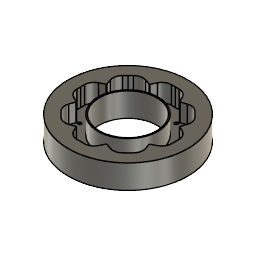
Nisip_Ghiveci (Autodesk Fusion 360 design; units mm, degrees)
part number: 2026-06-05-19-29-36-104
Autodesk Fusion 360 part; units mm, degrees
sketch "Sketch1" plane through (0, 0, 0) normal (0, 0, 1) x (1, 0, 0)
  arc A0 (13, 11.1068) -> (11.8, 12.3068) centre (11.8, 11.1068) ccw
  arc A1 (3.223, 0) -> (10.4161, 4.4986) centre (3.223, 8) ccw
  arc A2 (3.223, 0) -> (10.4161, 4.4986) centre (3.223, 8) ccw
  line L0 (10.5, 9.8068) -> (10.4144, 9.8073)
  arc A3 (13, 11.1068) -> (11.8, 12.3068) centre (11.8, 11.1068) ccw
  line L1 (10.5, 12.3068) -> (11.8, 12.3068)
  line L2 (10.5, 12.3068) -> (11.8, 12.3068)
  line L3 (13, 11.1068) -> (13, 10.9591)
  line L4 (13, 11.1068) -> (13, 10.9591)
  line L5 (12.4957, 8.7708) -> (10.4161, 4.4986)
  line L6 (10.2599, 10.1289) -> (10.5, 9.8068)
  line L7 (12.4957, 8.7708) -> (10.4161, 4.4986)
  arc A4 (12.4957, 8.7708) -> (13, 10.9591) centre (8, 10.9591) ccw
  line L8 (10.5, 12.3068) -> (-10.5, 12.3068)
  line L9 (0, 0) -> (3.223, 0)
  arc A5 (-13, 10.9591) -> (-12.4957, 8.7708) centre (-8, 10.9591) ccw
  line L10 (0, 0) -> (3.223, 0)
  line L11 (-12.4957, 8.7708) -> (-10.4161, 4.4986)
  line L12 (-3.223, 0) -> (0, 0)
  line L13 (-13, 11.1068) -> (-13, 10.9591)
  line L14 (-10.5, 12.3068) -> (-11.8, 12.3068)
  arc A6 (-11.8, 12.3068) -> (-13, 11.1068) centre (-11.8, 11.1068) ccw
  arc A7 (-10.4161, 4.4986) -> (-3.223, 0) centre (-3.223, 8) ccw
  arc A8 (12.4957, 8.7708) -> (13, 10.9591) centre (8, 10.9591) ccw
  circle A9 centre (-11.8, 11.1068) radius 0.875
  circle A10 centre (11.8, 11.1068) radius 0.875
  point P0 (-13, 12.3068)
  point P1 (13, 12.3068)
  dimension "d18" = 2.5
  dimension "d19" = 2.5
  dimension "d20" = 1.2
  dimension "d21" = 5
  dimension "d22" = 8
  dimension "d25" = 115.956
  dimension "d26" = 1.2
  dimension "d27" = 5
  dimension "d28" = 8
  dimension "d30" = 115.956
  dimension "d34" = 10.4144
  dimension "d35" = 9.8073
  dimension "d36" = 12.3068
  dimension "d37" = 13
  dimension "d38" = 13
  dimension "d39" = 8
  dimension "d40" = 12.3068
  dimension "d41" = 117.339
  dimension "d42" = 115.956
  dimension "d43" = 0.322
  dimension "d44" = 1.3477
  dimension "d45" = 1.75
  dimension "d46" = 1.75
  constraint horizontal L2
  constraint vertical L4
  constraint coincident L1.start L2.start
  constraint coincident L9.start L10.start
  constraint coincident P1 L2
  constraint coincident P1 L4
  constraint tangent A3 L2
  constraint tangent A3 L4
  constraint tangent L4 A4
  constraint tangent L5 A4
  constraint tangent A2 L9
  constraint tangent A2 L5
  constraint tangent A5 L13
  constraint tangent A5 L11
  constraint tangent L13 A6
  constraint tangent L14 A6
  constraint equal A4 A5
  constraint equal A3 A6
  constraint tangent L11 A7
  constraint tangent L12 A7
  constraint equal A2 A7
  constraint equal L4 L13
  constraint equal L2 L14
  constraint horizontal L8.end P0
  constraint collinear L2 L14
  constraint equal L9 L12
  constraint equal L5 L11
  constraint horizontal L1
  constraint vertical L3
  constraint tangent A0 L1
  constraint tangent A0 L3
  constraint tangent L3 A8
  constraint tangent L7 A8
  constraint tangent A1 L10
  constraint tangent A1 L7
  constraint tangent A1 L9
  constraint tangent A1 L5
  constraint tangent A0 L2
  constraint tangent L5 A8
  constraint tangent L4 A8
  constraint tangent A1 A2
  constraint collinear L5 L7
  constraint vertical L1.start L0.start
  constraint coincident L8.end L14.start
  constraint vertical P0 L13.start
  constraint concentric A6 A9
  constraint concentric A3 A10
  measures "d18" distance of L1.start P1
  measures "d19" distance of L1.start L0.start
  measures "d20" radius of A3
  measures "d21" radius of A4
  measures "d22" radius of A2
  measures "d25" angle of L5 L9
  measures "d26" radius of A0
  measures "d27" radius of A8
  measures "d28" radius of A1
  measures "d30" angle of L7 L10
  measures "d34" horizontal distance of L9.start L0.end
  measures "d35" vertical distance of L9.start L0.end
  measures "d36" distance of L9.start L8
  measures "d37" distance of L9.start L13
  measures "d38" distance of L9.start L4
  measures "d39" vertical distance of L9.start A1.centre
  measures "d40" distance of L9 L14
  measures "d41" angle of L5 L6
  measures "d42" angle of L11 L12
  measures "d43" vertical distance of L0.start L6.start
  measures "d44" distance of A4.centre L8
  measures "d45" diameter of A9
  measures "d46" diameter of A10
sketch "Sketch2" plane through (0, 0, 0) normal (0, 0, 1) x (1, 0, 0)
  line L0 (12.953, 8.964) -> (17.4443, 7.4136)
  circle A0 centre (11.793, 11.1078) radius 0.875
  line L1 (11.8637, 12.8755) -> (10.9445, 11.9563)
  arc A1 (17.4443, 7.4136) -> (25.7116, 9.3189) centre (20.0547, 14.9758) ccw
  arc A2 (10.9445, 11.9563) -> (10.9445, 10.2593) centre (11.793, 11.1078) ccw
  arc A3 (11.0489, 10.1548) -> (12.953, 8.964) centre (14.5845, 13.6903) ccw
  line L2 (27.9906, 11.5979) -> (30.2696, 13.877)
  line L3 (10.9445, 10.2593) -> (11.0489, 10.1548)
  circle A4 centre (28.4807, 27.7955) radius 0.875
  line L4 (27.9906, 11.5979) -> (30.2696, 13.877)
  arc A5 (30.6245, 26.6356) -> (29.4337, 28.5396) centre (25.8982, 25.0041) ccw
  line L5 (26.713, 27.7248) -> (27.6322, 28.644)
  arc A6 (30.2696, 13.877) -> (32.1749, 22.1442) centre (24.6128, 19.5338) ccw
  line L6 (25.7116, 9.3189) -> (27.9906, 11.5979)
  arc A7 (30.2696, 13.877) -> (32.1749, 22.1442) centre (24.6128, 19.5338) ccw
  arc A8 (30.6245, 26.6356) -> (29.4337, 28.5396) centre (25.8982, 25.0041) ccw
  line L7 (28.0833, 26.015) -> (28.4807, 25.957)
  line L8 (29.3293, 28.644) -> (29.4337, 28.5396)
  line L9 (29.3293, 28.644) -> (29.4337, 28.5396)
  arc A9 (29.3293, 28.644) -> (27.6322, 28.644) centre (28.4807, 27.7955) ccw
  line L10 (26.713, 27.7248) -> (11.8637, 12.8755)
  line L11 (26.713, 27.7248) -> (27.6322, 28.644)
  line L12 (30.6245, 26.6356) -> (32.1749, 22.1442)
  line L13 (28.4807, 25.957) -> (28.4199, 25.8969)
  arc A10 (29.3293, 28.644) -> (27.6322, 28.644) centre (28.4807, 27.7955) ccw
  line L14 (30.6245, 26.6356) -> (32.1749, 22.1442)
  line L15 (30.8154, 27.1043) -> (35.0875, 29.1838)
  circle A11 centre (28.4793, 27.7999) radius 0.875
  line L16 (27.2793, 29.0999) -> (27.2793, 27.7999)
  arc A12 (35.0875, 29.1838) -> (39.5861, 36.3769) centre (31.5861, 36.3769) ccw
  arc A13 (27.2793, 27.7999) -> (28.4793, 26.5999) centre (28.4793, 27.7999) ccw
  arc A14 (28.627, 26.5999) -> (30.8154, 27.1043) centre (28.627, 31.5999) ccw
  line L17 (39.5861, 39.5999) -> (39.5861, 42.823)
  line L18 (28.4793, 26.5999) -> (28.627, 26.5999)
  circle A15 centre (28.4793, 51.3999) radius 0.875
  line L19 (39.5861, 39.5999) -> (39.5861, 42.823)
  arc A16 (30.8154, 52.0956) -> (28.627, 52.5999) centre (28.627, 47.5999) ccw
  line L20 (27.2793, 50.0999) -> (27.2793, 51.3999)
  arc A17 (39.5861, 42.823) -> (35.0875, 50.0161) centre (31.5861, 42.823) ccw
  line L21 (39.5861, 36.3769) -> (39.5861, 39.5999)
  arc A18 (39.5861, 42.823) -> (35.0875, 50.0161) centre (31.5861, 42.823) ccw
  arc A19 (30.8154, 52.0956) -> (28.627, 52.5999) centre (28.627, 47.5999) ccw
  line L22 (29.4573, 49.8599) -> (29.7793, 50.0999)
  line L23 (28.4793, 52.5999) -> (28.627, 52.5999)
  line L24 (28.4793, 52.5999) -> (28.627, 52.5999)
  arc A20 (28.4793, 52.5999) -> (27.2793, 51.3999) centre (28.4793, 51.3999) ccw
  line L25 (27.2793, 50.0999) -> (27.2793, 29.0999)
  line L26 (27.2793, 50.0999) -> (27.2793, 51.3999)
  line L27 (30.8154, 52.0956) -> (35.0875, 50.0161)
  line L28 (29.7793, 50.0999) -> (29.7788, 50.0144)
  arc A21 (28.4793, 52.5999) -> (27.2793, 51.3999) centre (28.4793, 51.3999) ccw
  line L29 (30.8154, 52.0956) -> (35.0875, 50.0161)
  line L30 (3.1934, 79.2434) -> (-0.0296, 79.2434)
  line L31 (-10.5296, 66.9366) -> (-11.8296, 66.9366)
  line L32 (-10.5296, 66.9366) -> (10.4704, 66.9366)
  arc A22 (-3.2527, 79.2434) -> (-10.4458, 74.7448) centre (-3.2527, 71.2434) ccw
  arc A23 (-13.0296, 68.1366) -> (-11.8296, 66.9366) centre (-11.8296, 68.1366) ccw
  line L33 (-12.5253, 70.4727) -> (-10.4458, 74.7448)
  line L34 (-13.0296, 68.1366) -> (-13.0296, 68.2843)
  arc A24 (-12.5253, 70.4727) -> (-13.0296, 68.2843) centre (-8.0296, 68.2843) ccw
  line L35 (11.8455, 66.3703) -> (10.9263, 67.2895)
  line L36 (13.5553, 67.7406) -> (13.6133, 68.1381)
  arc A25 (10.9263, 68.9866) -> (10.9263, 67.2895) centre (11.7748, 68.1381) ccw
  arc A26 (25.6933, 69.9269) -> (17.4261, 71.8322) centre (20.0365, 64.2701) ccw
  line L37 (13.6133, 68.1381) -> (13.6734, 68.0772)
  line L38 (10.9263, 68.9866) -> (11.0307, 69.091)
  arc A27 (11.7704, 66.9366) -> (12.9704, 68.1366) centre (11.7704, 68.1366) ccw
  line L39 (12.466, 70.4727) -> (10.3865, 74.7448)
  line L40 (11.8455, 66.3703) -> (10.9263, 67.2895)
  arc A28 (12.9704, 68.2843) -> (12.466, 70.4727) centre (7.9704, 68.2843) ccw
  arc A29 (10.3865, 74.7448) -> (3.1934, 79.2434) centre (3.1934, 71.2434) ccw
  line L41 (10.4704, 66.9366) -> (11.7704, 66.9366)
  line L42 (12.9347, 70.2818) -> (17.4261, 71.8322)
  arc A30 (25.6933, 69.9269) -> (17.4261, 71.8322) centre (20.0365, 64.2701) ccw
  circle A31 centre (11.7748, 68.1381) radius 0.875
  circle A32 centre (11.7704, 68.1366) radius 0.875
  arc A33 (12.9347, 70.2818) -> (11.0307, 69.091) centre (14.5663, 65.5555) ccw
  line L43 (-0.0296, 79.2434) -> (-3.2527, 79.2434)
  arc A34 (-3.2527, 79.2434) -> (-10.4458, 74.7448) centre (-3.2527, 71.2434) ccw
  circle A35 centre (-11.8296, 68.1366) radius 0.875
  line L44 (27.9724, 67.6479) -> (25.6933, 69.9269)
  line L45 (11.8455, 66.3703) -> (26.6948, 51.521)
  circle A36 centre (28.4625, 51.4503) radius 0.875
  arc A37 (32.1567, 57.1016) -> (30.2514, 65.3689) centre (24.5945, 59.712) ccw
  arc A38 (29.4155, 50.7062) -> (30.6063, 52.6103) centre (25.88, 54.2418) ccw
  line L46 (27.9724, 67.6479) -> (25.6933, 69.9269)
  line L47 (26.6948, 51.521) -> (27.614, 50.6018)
  arc A39 (27.614, 50.6018) -> (29.3111, 50.6018) centre (28.4625, 51.4503) ccw
  line L48 (30.6063, 52.6103) -> (32.1567, 57.1016)
  arc A40 (12.9347, 70.2818) -> (11.0307, 69.091) centre (14.5663, 65.5555) ccw
  arc A41 (10.9263, 68.9866) -> (10.9263, 67.2895) centre (11.7748, 68.1381) ccw
  line L49 (12.9347, 70.2818) -> (17.4261, 71.8322)
  line L50 (12.9704, 68.1366) -> (12.9704, 68.2843)
  line L51 (10.9263, 68.9866) -> (11.0307, 69.091)
  line L52 (-12.5253, 70.4727) -> (-10.4458, 74.7448)
  arc A42 (-12.5253, 70.4727) -> (-13.0296, 68.2843) centre (-8.0296, 68.2843) ccw
  line L53 (-10.5296, 69.4366) -> (-10.4441, 69.4361)
  line L54 (-0.0296, 79.2434) -> (-3.2527, 79.2434)
  arc A43 (-13.0296, 68.1366) -> (-11.8296, 66.9366) centre (-11.8296, 68.1366) ccw
  line L55 (-10.5296, 66.9366) -> (-11.8296, 66.9366)
  line L56 (29.3111, 50.6018) -> (29.4155, 50.7062)
  line L57 (30.2514, 65.3689) -> (27.9724, 67.6479)
  line L58 (-13.0296, 68.1366) -> (-13.0296, 68.2843)
  line L59 (-10.2896, 69.1146) -> (-10.5296, 69.4366)
  line L60 (12.9689, 11.1314) -> (12.9689, 10.9837)
  line L61 (12.9689, 11.1314) -> (12.9689, 10.9837)
  line L62 (-0.0311, 0.0246) -> (3.192, 0.0246)
  arc A44 (12.4646, 8.7953) -> (12.9689, 10.9837) centre (7.9689, 10.9837) ccw
  line L63 (12.4646, 8.7953) -> (10.385, 4.5232)
  arc A45 (12.9689, 11.1314) -> (11.7689, 12.3314) centre (11.7689, 11.1314) ccw
  line L64 (10.4689, 9.8314) -> (10.3834, 9.8319)
  line L65 (10.4689, 12.3314) -> (11.7689, 12.3314)
  arc A46 (3.192, 0.0246) -> (10.385, 4.5232) centre (3.192, 8.0246) ccw
  line L66 (-11.9244, 66.3925) -> (-11.0052, 67.3117)
  arc A47 (-11.1097, 69.1132) -> (-13.0137, 70.304) centre (-14.6452, 65.5777) ccw
  line L67 (10.4689, 12.3314) -> (-10.5311, 12.3314)
  arc A48 (-11.0052, 67.3117) -> (-11.0052, 69.0088) centre (-11.8537, 68.1602) ccw
  line L68 (-11.0052, 69.0088) -> (-11.1097, 69.1132)
  arc A49 (-10.4472, 4.5232) -> (-3.2541, 0.0246) centre (-3.2541, 8.0246) ccw
  line L69 (-28.0513, 67.6701) -> (-30.3303, 65.3911)
  line L70 (-28.0513, 67.6701) -> (-30.3303, 65.3911)
  line L71 (-26.7737, 51.5432) -> (-11.9244, 66.3925)
  line L72 (10.4689, 12.3314) -> (11.7689, 12.3314)
  line L73 (-3.2541, 0.0246) -> (-0.0311, 0.0246)
  arc A50 (3.192, 0.0246) -> (10.385, 4.5232) centre (3.192, 8.0246) ccw
  circle A51 centre (11.7689, 11.1314) radius 0.875
  line L74 (-11.9062, 12.8977) -> (-10.987, 11.9785)
  line L75 (-13.616, 11.5274) -> (-13.674, 11.13)
  arc A52 (-12.9955, 8.9862) -> (-11.0914, 10.177) centre (-14.627, 13.7125) ccw
  line L76 (-10.987, 10.2814) -> (-11.0914, 10.177)
  arc A53 (-11.8311, 12.3314) -> (-13.0311, 11.1314) centre (-11.8311, 11.1314) ccw
  arc A54 (-13.0311, 10.9837) -> (-12.5267, 8.7953) centre (-8.0311, 10.9837) ccw
  arc A55 (-12.9955, 8.9862) -> (-11.0914, 10.177) centre (-14.627, 13.7125) ccw
  arc A56 (-25.7541, 9.3411) -> (-17.4868, 7.4358) centre (-20.0972, 14.9979) ccw
  line L77 (-10.5311, 12.3314) -> (-11.8311, 12.3314)
  line L78 (-12.9955, 8.9862) -> (-17.4868, 7.4358)
  arc A57 (-10.987, 10.2814) -> (-10.987, 11.9785) centre (-11.8355, 11.13) ccw
  arc A58 (-10.987, 10.2814) -> (-10.987, 11.9785) centre (-11.8355, 11.13) ccw
  line L79 (-12.9955, 8.9862) -> (-17.4868, 7.4358)
  line L80 (-10.987, 10.2814) -> (-11.0914, 10.177)
  line L81 (-39.6468, 39.6681) -> (-39.6468, 36.445)
  line L82 (-26.7555, 27.747) -> (-27.6747, 28.6662)
  line L83 (-29.84, 29.1681) -> (-29.8395, 29.2536)
  line L84 (-30.3121, 13.8991) -> (-28.0331, 11.6201)
  line L85 (-29.3718, 28.6662) -> (-29.4762, 28.5618)
  arc A59 (-32.2174, 22.1664) -> (-30.3121, 13.8991) centre (-24.6553, 19.556) ccw
  arc A60 (-30.8761, 27.1724) -> (-28.6877, 26.6681) centre (-28.6877, 31.6681) ccw
  arc A61 (-39.6468, 36.445) -> (-35.1482, 29.252) centre (-31.6468, 36.445) ccw
  circle A62 centre (-28.5232, 27.8177) radius 0.875
  line L86 (-30.667, 26.6577) -> (-32.2174, 22.1664)
  arc A63 (-29.4762, 28.5618) -> (-30.667, 26.6577) centre (-25.9407, 25.0262) ccw
  arc A64 (-27.6747, 28.6662) -> (-29.3718, 28.6662) centre (-28.5232, 27.8177) ccw
  line L87 (-27.34, 29.1681) -> (-27.34, 27.8681)
  circle A65 centre (-11.8311, 11.1314) radius 0.875
  circle A66 centre (-11.8537, 68.1602) radius 0.875
  line L88 (-25.7723, 69.9491) -> (-28.0513, 67.6701)
  line L89 (-30.6852, 52.6325) -> (-32.2356, 57.1238)
  line L90 (-39.6468, 42.8911) -> (-39.6468, 39.6681)
  arc A67 (-17.505, 71.8544) -> (-25.7723, 69.9491) centre (-20.1154, 64.2923) ccw
  line L91 (-13.0137, 70.304) -> (-17.505, 71.8544)
  line L92 (-27.34, 29.1681) -> (-27.34, 50.1681)
  arc A68 (12.9689, 11.1314) -> (11.7689, 12.3314) centre (11.7689, 11.1314) ccw
  line L93 (12.4646, 8.7953) -> (10.385, 4.5232)
  arc A69 (12.4646, 8.7953) -> (12.9689, 10.9837) centre (7.9689, 10.9837) ccw
  line L94 (-0.0311, 0.0246) -> (3.192, 0.0246)
  line L95 (10.2288, 10.1534) -> (10.4689, 9.8314)
  arc A70 (-30.3303, 65.3911) -> (-32.2356, 57.1238) centre (-24.6735, 59.7342) ccw
  line L96 (-28.54, 52.6681) -> (-28.6877, 52.6681)
  line L97 (-28.144, 53.253) -> (-28.5415, 53.311)
  line L98 (-30.6852, 52.6325) -> (-32.2356, 57.1238)
  line L99 (-28.5415, 53.311) -> (-28.4806, 53.3711)
  arc A71 (-30.3303, 65.3911) -> (-32.2356, 57.1238) centre (-24.6735, 59.7342) ccw
  arc A72 (-35.1482, 50.0842) -> (-39.6468, 42.8911) centre (-31.6468, 42.8911) ccw
  line L100 (-29.39, 50.624) -> (-29.4944, 50.7284)
  line L101 (-27.34, 50.1681) -> (-27.34, 51.4681)
  line L102 (-26.7737, 51.5432) -> (-27.6929, 50.624)
  arc A73 (-30.6852, 52.6325) -> (-29.4944, 50.7284) centre (-25.9589, 54.264) ccw
  circle A74 centre (-28.54, 51.4681) radius 0.875
  arc A75 (-25.7541, 9.3411) -> (-17.4868, 7.4358) centre (-20.0972, 14.9979) ccw
  line L103 (-11.9062, 12.8977) -> (-10.987, 11.9785)
  line L104 (-13.674, 11.13) -> (-13.7341, 11.1908)
  circle A76 centre (-11.8355, 11.13) radius 0.875
  line L105 (-13.0311, 11.1314) -> (-13.0311, 10.9837)
  line L106 (-12.5267, 8.7953) -> (-10.4472, 4.5232)
  circle A77 centre (-28.54, 27.8681) radius 0.875
  arc A78 (-28.54, 26.6681) -> (-27.34, 27.8681) centre (-28.54, 27.8681) ccw
  arc A79 (-39.6468, 36.445) -> (-35.1482, 29.252) centre (-31.6468, 36.445) ccw
  line L107 (-28.0331, 11.6201) -> (-25.7541, 9.3411)
  line L108 (-30.8761, 27.1724) -> (-35.1482, 29.252)
  circle A80 centre (-28.5415, 51.4725) radius 0.875
  arc A81 (-29.39, 50.624) -> (-27.6929, 50.624) centre (-28.5415, 51.4725) ccw
  line L109 (-30.8761, 52.1637) -> (-35.1482, 50.0842)
  line L110 (-28.54, 26.6681) -> (-28.6877, 26.6681)
  line L111 (-29.39, 50.624) -> (-29.4944, 50.7284)
  line L112 (-30.8761, 27.1724) -> (-35.1482, 29.252)
  arc A82 (-28.54, 26.6681) -> (-27.34, 27.8681) centre (-28.54, 27.8681) ccw
  line L113 (-29.518, 29.4082) -> (-29.84, 29.1681)
  arc A83 (-28.6877, 52.6681) -> (-30.8761, 52.1637) centre (-28.6877, 47.6681) ccw
  arc A84 (-30.8761, 27.1724) -> (-28.6877, 26.6681) centre (-28.6877, 31.6681) ccw
  line L114 (-28.54, 26.6681) -> (-28.6877, 26.6681)
  line L115 (-26.7737, 51.5432) -> (-27.6929, 50.624)
  line L116 (-28.0331, 11.6201) -> (-25.7541, 9.3411)
  line L117 (-11.9062, 12.8977) -> (-26.7555, 27.747)
  arc A85 (-27.34, 51.4681) -> (-28.54, 52.6681) centre (-28.54, 51.4681) ccw
  arc A86 (-30.6852, 52.6325) -> (-29.4944, 50.7284) centre (-25.9589, 54.264) ccw
  line L118 (-39.6468, 39.6681) -> (-39.6468, 36.445)
  arc A87 (-29.39, 50.624) -> (-27.6929, 50.624) centre (-28.5415, 51.4725) ccw
  line L119 (-27.34, 29.1681) -> (-27.34, 27.8681)
  line L120 (11.2792, 66.9366) -> (-11.3399, 12.3314)
  line L121 (-11.3399, 12.3314) -> (-11.3316, 12.3514)
  line L122 (11.3196, 12.3314) -> (-11.3803, 66.9366)
  circle A88 centre (-0.0304, 39.634) radius 25
  circle A89 centre (-0.0304, 39.634) radius 50
  circle A90 centre (-0.0304, 39.634) radius 24
  point P0 (27.9906, 11.5979)
  point P1 (10.096, 11.1078)
  point P2 (28.4807, 29.4926)
  point P3 (27.9906, 11.5979)
  point P4 (39.5861, 39.5999)
  point P5 (27.2793, 26.5999)
  point P6 (27.2793, 52.5999)
  point P7 (39.5861, 39.5999)
  point P8 (-13.0296, 66.9366)
  point P9 (-0.0296, 79.2434)
  point P10 (-0.0296, 79.2434)
  point P11 (12.9704, 66.9366)
  point P12 (27.9724, 67.6479)
  point P13 (28.4625, 49.7533)
  point P14 (27.9724, 67.6479)
  point P15 (10.0777, 68.1381)
  point P16 (-28.5232, 29.5147)
  point P17 (-28.0331, 11.6201)
  point P18 (-10.1385, 11.13)
  point P19 (-28.0331, 11.6201)
  point P20 (-27.34, 26.6681)
  point P21 (-39.6468, 39.6681)
  point P22 (-39.6468, 39.6681)
  point P23 (-27.34, 52.6681)
  point P24 (-0.0607, 79.268)
  point P25 (-28.0513, 67.6701)
  point P26 (-10.1567, 68.1602)
  point P27 (-28.0513, 67.6701)
  point P28 (-28.5415, 49.7755)
  point P29 (12.9689, 12.3314)
  point P30 (-0.0311, 0.0246)
  point P31 (-0.0311, 0.0246)
  point P32 (-13.0311, 12.3314)
  dimension "d49" = 2.5
  dimension "d50" = 2.5
  dimension "d51" = 1.2
  dimension "d52" = 5
  dimension "d53" = 8
  dimension "d54" = 115.956
  dimension "d55" = 1.2
  dimension "d56" = 5
  dimension "d57" = 8
  dimension "d58" = 115.956
  dimension "d61" = 12.3068
  dimension "d62" = 13
  dimension "d63" = 13
  dimension "d65" = 12.3068
  dimension "d66" = 117.339
  dimension "d67" = 115.956
  dimension "d69" = 1.3477
  dimension "d70" = 1.75
  dimension "d71" = 1.75
  dimension "d72" = 2.5
  dimension "d73" = 2.5
  dimension "d74" = 1.2
  dimension "d75" = 5
  dimension "d76" = 8
  dimension "d77" = 115.956
  dimension "d78" = 1.2
  dimension "d79" = 5
  dimension "d80" = 8
  dimension "d81" = 115.956
  dimension "d84" = 12.3068
  dimension "d85" = 13
  dimension "d86" = 13
  dimension "d88" = 12.3068
  dimension "d89" = 117.339
  dimension "d90" = 115.956
  dimension "d92" = 1.3477
  dimension "d93" = 1.75
  dimension "d94" = 1.75
  dimension "d95" = 2.5
  dimension "d96" = 2.5
  dimension "d97" = 1.2
  dimension "d98" = 5
  dimension "d99" = 8
  dimension "d100" = 115.956
  dimension "d101" = 1.2
  dimension "d102" = 5
  dimension "d103" = 8
  dimension "d104" = 115.956
  dimension "d105" = 12.3068
  dimension "d106" = 13
  dimension "d107" = 13
  dimension "d108" = 12.3068
  dimension "d109" = 117.339
  dimension "d110" = 115.956
  dimension "d111" = 1.3477
  dimension "d112" = 1.75
  dimension "d113" = 1.75
  dimension "d114" = 2.5
  dimension "d115" = 2.5
  dimension "d116" = 1.2
  dimension "d117" = 5
  dimension "d118" = 8
  dimension "d119" = 115.956
  dimension "d120" = 1.2
  dimension "d121" = 5
  dimension "d122" = 8
  dimension "d123" = 115.956
  dimension "d124" = 12.3068
  dimension "d125" = 13
  dimension "d126" = 13
  dimension "d127" = 12.3068
  dimension "d128" = 117.339
  dimension "d129" = 115.956
  dimension "d130" = 1.3477
  dimension "d131" = 1.75
  dimension "d132" = 1.75
  dimension "d133" = 2.5
  dimension "d134" = 2.5
  dimension "d135" = 1.2
  dimension "d136" = 5
  dimension "d137" = 8
  dimension "d138" = 115.956
  dimension "d139" = 1.2
  dimension "d140" = 5
  dimension "d141" = 8
  dimension "d142" = 115.956
  dimension "d143" = 12.3068
  dimension "d144" = 13
  dimension "d145" = 13
  dimension "d146" = 12.3068
  dimension "d147" = 117.339
  dimension "d148" = 115.956
  dimension "d149" = 1.3477
  dimension "d150" = 1.75
  dimension "d151" = 1.75
  dimension "d152" = 2.5
  dimension "d153" = 2.5
  dimension "d154" = 1.2
  dimension "d155" = 5
  dimension "d156" = 8
  dimension "d157" = 115.956
  dimension "d158" = 1.2
  dimension "d159" = 5
  dimension "d160" = 8
  dimension "d161" = 115.956
  dimension "d162" = 12.3068
  dimension "d163" = 13
  dimension "d164" = 13
  dimension "d165" = 12.3068
  dimension "d166" = 117.339
  dimension "d167" = 115.956
  dimension "d168" = 1.3477
  dimension "d169" = 1.75
  dimension "d170" = 1.75
  dimension "d171" = 2.5
  dimension "d172" = 2.5
  dimension "d173" = 1.2
  dimension "d174" = 5
  dimension "d175" = 8
  dimension "d176" = 115.956
  dimension "d177" = 1.2
  dimension "d178" = 5
  dimension "d179" = 8
  dimension "d180" = 115.956
  dimension "d181" = 12.3068
  dimension "d182" = 13
  dimension "d183" = 13
  dimension "d184" = 12.3068
  dimension "d185" = 117.339
  dimension "d186" = 115.956
  dimension "d187" = 1.3477
  dimension "d188" = 1.75
  dimension "d189" = 1.75
  dimension "d190" = 2.5
  dimension "d191" = 2.5
  dimension "d192" = 1.2
  dimension "d193" = 5
  dimension "d194" = 8
  dimension "d195" = 115.956
  dimension "d196" = 1.2
  dimension "d197" = 5
  dimension "d198" = 8
  dimension "d199" = 115.956
  dimension "d200" = 12.3068
  dimension "d201" = 13
  dimension "d202" = 13
  dimension "d203" = 12.3068
  dimension "d204" = 117.339
  dimension "d205" = 115.956
  dimension "d206" = 1.3477
  dimension "d207" = 1.75
  dimension "d208" = 1.75
  dimension "d211" = 50
  dimension "d212" = 100
  dimension "d213" = -1
  constraint coincident L5.start L10.start
  constraint coincident P3 P0
  constraint coincident P2 L5
  constraint coincident P2 L8
  constraint tangent L5 A9
  constraint tangent L8 A9
  constraint tangent A5 L8
  constraint tangent A5 L14
  constraint tangent L4 A6
  constraint tangent A6 L14
  constraint tangent A3 L3
  constraint tangent L0 A3
  constraint tangent A2 L3
  constraint tangent L1 A2
  constraint equal A3 A5
  constraint equal A2 A9
  constraint tangent L0 A1
  constraint tangent A1 L6
  constraint equal A1 A6
  constraint equal L3 L8
  constraint equal L1 L5
  constraint collinear L1 L5
  constraint equal L4 L6
  constraint equal L0 L14
  constraint tangent L11 A10
  constraint tangent L9 A10
  constraint tangent A8 L9
  constraint tangent A8 L12
  constraint tangent L2 A7
  constraint tangent A7 L12
  constraint tangent L4 A7
  constraint tangent A7 L14
  constraint tangent L5 A10
  constraint tangent A8 L14
  constraint tangent A8 L8
  constraint tangent A6 A7
  constraint collinear L12 L14
  constraint coincident L1.start L10.end
  constraint concentric A0 A2
  constraint concentric A4 A9
  constraint coincident L20.start L25.start
  constraint coincident P7 P4
  constraint coincident P6 L20
  constraint coincident P6 L23
  constraint tangent L20 A20
  constraint tangent L23 A20
  constraint tangent A16 L23
  constraint tangent A16 L29
  constraint tangent L19 A17
  constraint tangent A17 L29
  constraint tangent A14 L18
  constraint tangent L15 A14
  constraint tangent A13 L18
  constraint tangent L16 A13
  constraint equal A14 A16
  constraint equal A13 A20
  constraint tangent L15 A12
  constraint tangent A12 L21
  constraint equal A12 A17
  constraint equal L18 L23
  constraint equal L16 L20
  constraint collinear L16 L20
  constraint equal L19 L21
  constraint equal L15 L29
  constraint tangent L26 A21
  constraint tangent L24 A21
  constraint tangent A19 L24
  constraint tangent A19 L27
  constraint tangent L17 A18
  constraint tangent A18 L27
  constraint tangent L19 A18
  constraint tangent A18 L29
  constraint tangent L20 A21
  constraint tangent A19 L29
  constraint tangent A19 L23
  constraint tangent A17 A18
  constraint collinear L27 L29
  constraint coincident L16.start L25.end
  constraint concentric A11 A13
  constraint concentric A15 A20
  constraint coincident L35.start L40.start
  constraint coincident P14 P12
  constraint coincident P15 L35
  constraint coincident P15 L38
  constraint tangent L35 A41
  constraint tangent L38 A41
  constraint tangent L38 A33
  constraint tangent A33 L49
  constraint tangent A30 L46
  constraint tangent A30 L49
  constraint tangent A38 L56
  constraint tangent A38 L48
  constraint tangent A39 L56
  constraint tangent L47 A39
  constraint equal A33 A38
  constraint equal A39 A41
  constraint tangent A37 L48
  constraint tangent A37 L57
  constraint equal A30 A37
  constraint equal L38 L56
  constraint equal L35 L47
  constraint collinear L35 L47
  constraint equal L46 L57
  constraint equal L48 L49
  constraint tangent A25 L40
  constraint tangent A25 L51
  constraint tangent A40 L51
  constraint tangent L42 A40
  constraint tangent A26 L44
  constraint tangent A26 L42
  constraint tangent A26 L46
  constraint tangent A26 L49
  constraint tangent L35 A25
  constraint tangent A40 L49
  constraint tangent L38 A40
  constraint tangent A26 A30
  constraint collinear L42 L49
  constraint coincident L45.end L47.start
  constraint concentric A36 A39
  constraint concentric A31 A41
  constraint coincident L31.start L32.start
  constraint coincident P10 P9
  constraint coincident P8 L55
  constraint coincident P8 L58
  constraint tangent A23 L55
  constraint tangent A23 L58
  constraint tangent A42 L58
  constraint tangent L33 A42
  constraint tangent A34 L54
  constraint tangent L33 A34
  constraint tangent A28 L50
  constraint tangent L39 A28
  constraint tangent A27 L50
  constraint tangent A27 L41
  constraint equal A28 A42
  constraint equal A23 A27
  constraint tangent L39 A29
  constraint tangent L30 A29
  constraint equal A29 A34
  constraint equal L50 L58
  constraint equal L41 L55
  constraint collinear L41 L55
  constraint equal L30 L54
  constraint equal L33 L39
  constraint tangent L31 A43
  constraint tangent L34 A43
  constraint tangent L34 A24
  constraint tangent A24 L52
  constraint tangent A22 L43
  constraint tangent A22 L52
  constraint tangent A22 L54
  constraint tangent A22 L33
  constraint tangent A43 L55
  constraint tangent L33 A24
  constraint tangent A24 L58
  constraint tangent A22 A34
  constraint collinear L33 L52
  constraint coincident L32.end L41.start
  constraint concentric A27 A32
  constraint concentric A23 A35
  constraint coincident L71.start L102.start
  constraint coincident P27 P25
  constraint coincident P28 L102
  constraint coincident P28 L100
  constraint tangent L102 A81
  constraint tangent L100 A81
  constraint tangent L100 A73
  constraint tangent L98 A73
  constraint tangent L70 A70
  constraint tangent A70 L98
  constraint tangent A47 L68
  constraint tangent A47 L91
  constraint tangent A48 L68
  constraint tangent L66 A48
  constraint equal A47 A73
  constraint equal A48 A81
  constraint tangent A67 L91
  constraint tangent L88 A67
  constraint equal A67 A70
  constraint equal L68 L100
  constraint equal L66 L102
  constraint collinear L66 L102
  constraint equal L70 L88
  constraint equal L91 L98
  constraint tangent L115 A87
  constraint tangent L111 A87
  constraint tangent L111 A86
  constraint tangent L89 A86
  constraint tangent L69 A71
  constraint tangent L89 A71
  constraint tangent L70 A71
  constraint tangent L98 A71
  constraint tangent L102 A87
  constraint tangent L98 A86
  constraint tangent L100 A86
  constraint tangent A70 A71
  constraint collinear L89 L98
  constraint coincident L66.start L71.end
  constraint concentric A48 A66
  constraint concentric A80 A81
  constraint coincident L87.start L92.start
  constraint coincident P22 P21
  constraint coincident P20 L119
  constraint coincident P20 L110
  constraint tangent A82 L119
  constraint tangent L110 A82
  constraint tangent L110 A84
  constraint tangent L112 A84
  constraint tangent A61 L118
  constraint tangent A61 L112
  constraint tangent L96 A83
  constraint tangent L109 A83
  constraint tangent L96 A85
  constraint tangent L101 A85
  constraint equal A83 A84
  constraint equal A82 A85
  constraint tangent A72 L109
  constraint tangent L90 A72
  constraint equal A61 A72
  constraint equal L96 L110
  constraint equal L101 L119
  constraint collinear L101 L119
  constraint equal L90 L118
  constraint equal L109 L112
  constraint tangent L87 A78
  constraint tangent A78 L114
  constraint tangent A60 L114
  constraint tangent A60 L108
  constraint tangent L81 A79
  constraint tangent A79 L108
  constraint tangent A79 L118
  constraint tangent A79 L112
  constraint tangent A78 L119
  constraint tangent A60 L112
  constraint tangent A60 L110
  constraint tangent A61 A79
  constraint collinear L108 L112
  constraint coincident L92.end L101.start
  constraint concentric A74 A85
  constraint concentric A77 A82
  constraint coincident L74.start L103.start
  constraint coincident P19 P17
  constraint coincident P18 L103
  constraint coincident P18 L80
  constraint tangent A58 L103
  constraint tangent A58 L80
  constraint tangent A52 L80
  constraint tangent A52 L78
  constraint tangent A56 L116
  constraint tangent A56 L78
  constraint tangent L85 A63
  constraint tangent L86 A63
  constraint tangent L85 A64
  constraint tangent L82 A64
  constraint equal A52 A63
  constraint equal A58 A64
  constraint tangent A59 L86
  constraint tangent L84 A59
  constraint equal A56 A59
  constraint equal L80 L85
  constraint equal L82 L103
  constraint collinear L82 L103
  constraint equal L84 L116
  constraint equal L78 L86
  constraint tangent L74 A57
  constraint tangent L76 A57
  constraint tangent L76 A55
  constraint tangent A55 L79
  constraint tangent A75 L107
  constraint tangent L79 A75
  constraint tangent A75 L116
  constraint tangent L78 A75
  constraint tangent A57 L103
  constraint tangent A55 L78
  constraint tangent A55 L80
  constraint tangent A56 A75
  constraint collinear L78 L79
  constraint coincident L82.start L117.end
  constraint concentric A62 A64
  constraint concentric A58 A76
  constraint coincident L65.start L67.start
  constraint coincident P31 P30
  constraint coincident P29 L72
  constraint coincident P29 L60
  constraint tangent A45 L72
  constraint tangent L60 A45
  constraint tangent L60 A69
  constraint tangent L93 A69
  constraint tangent A50 L94
  constraint tangent A50 L93
  constraint tangent A54 L105
  constraint tangent A54 L106
  constraint tangent A53 L105
  constraint tangent A53 L77
  constraint equal A54 A69
  constraint equal A45 A53
  constraint tangent A49 L106
  constraint tangent A49 L73
  constraint equal A49 A50
  constraint equal L60 L105
  constraint equal L72 L77
  constraint collinear L72 L77
  constraint equal L73 L94
  constraint equal L93 L106
  constraint tangent L65 A68
  constraint tangent L61 A68
  constraint tangent L61 A44
  constraint tangent A44 L63
  constraint tangent L62 A46
  constraint tangent L63 A46
  constraint tangent A46 L94
  constraint tangent A46 L93
  constraint tangent L72 A68
  constraint tangent A44 L93
  constraint tangent L60 A44
  constraint tangent A46 A50
  constraint collinear L63 L93
  constraint coincident L67.end L77.start
  constraint concentric A53 A65
  constraint concentric A45 A51
  constraint coincident L40 L120.start
  constraint coincident L41 L120.start
  constraint coincident L103 L120.end
  constraint coincident L77 L120.end
  constraint coincident L120 L121.end
  constraint coincident L72 L122.start
  constraint coincident L1 L122.start
  constraint coincident L31 L122.end
  constraint coincident L66 L122.end
  constraint midpoint L120 A88.centre
  constraint concentric A88 A89
  measures "d49" distance of L5.start P2
  measures "d50" distance of L5.start L7.end
  measures "d51" radius of A9
  measures "d52" radius of A5
  measures "d53" radius of A6
  measures "d54" angle of L4 L14
  measures "d55" radius of A10
  measures "d56" radius of A8
  measures "d57" radius of A7
  measures "d58" angle of L2 L12
  measures "d61" distance of P3 L10
  measures "d62" distance of P3 L3
  measures "d63" distance of P3 L8
  measures "d65" distance of L1 L4
  measures "d66" angle of L7 L14
  measures "d67" angle of L0 L6
  measures "d69" distance of A5.centre L10
  measures "d70" diameter of A0
  measures "d71" diameter of A4
  measures "d72" distance of L20.start P6
  measures "d73" distance of L20.start L22.end
  measures "d74" radius of A20
  measures "d75" radius of A16
  measures "d76" radius of A17
  measures "d77" angle of L19 L29
  measures "d78" radius of A21
  measures "d79" radius of A19
  measures "d80" radius of A18
  measures "d81" angle of L17 L27
  measures "d84" distance of P7 L25
  measures "d85" distance of P7 L18
  measures "d86" distance of P7 L23
  measures "d88" distance of L16 L19
  measures "d89" angle of L22 L29
  measures "d90" angle of L15 L21
  measures "d92" distance of A16.centre L25
  measures "d93" diameter of A11
  measures "d94" diameter of A15
  measures "d95" distance of L35.start P15
  measures "d96" distance of L35.start L36.end
  measures "d97" radius of A41
  measures "d98" radius of A33
  measures "d99" radius of A30
  measures "d100" angle of L46 L49
  measures "d101" radius of A25
  measures "d102" radius of A40
  measures "d103" radius of A26
  measures "d104" angle of L42 L44
  measures "d105" distance of P14 L45
  measures "d106" distance of P14 L56
  measures "d107" distance of P14 L38
  measures "d108" distance of L46 L47
  measures "d109" angle of L36 L49
  measures "d110" angle of L48 L57
  measures "d111" distance of A33.centre L45
  measures "d112" diameter of A36
  measures "d113" diameter of A31
  measures "d114" distance of P8 L31.start
  measures "d115" distance of L53.start L31.start
  measures "d116" radius of A23
  measures "d117" radius of A42
  measures "d118" radius of A34
  measures "d119" angle of L33 L54
  measures "d120" radius of A43
  measures "d121" radius of A24
  measures "d122" radius of A22
  measures "d123" angle of L43 L52
  measures "d124" distance of P10 L32
  measures "d125" distance of P10 L50
  measures "d126" distance of P10 L58
  measures "d127" distance of L41 L54
  measures "d128" angle of L33 L59
  measures "d129" angle of L30 L39
  measures "d130" distance of A24.centre L32
  measures "d131" diameter of A32
  measures "d132" diameter of A35
  measures "d133" distance of L71.start P28
  measures "d134" distance of L71.start L97.end
  measures "d135" radius of A81
  measures "d136" radius of A73
  measures "d137" radius of A70
  measures "d138" angle of L70 L98
  measures "d139" radius of A87
  measures "d140" radius of A86
  measures "d141" radius of A71
  measures "d142" angle of L69 L89
  measures "d143" distance of P27 L71
  measures "d144" distance of P27 L68
  measures "d145" distance of P27 L100
  measures "d146" distance of L66 L70
  measures "d147" angle of L97 L98
  measures "d148" angle of L88 L91
  measures "d149" distance of A73.centre L71
  measures "d150" diameter of A66
  measures "d151" diameter of A80
  measures "d152" distance of P20 L87.start
  measures "d153" distance of L83.start L87.start
  measures "d154" radius of A82
  measures "d155" radius of A84
  measures "d156" radius of A61
  measures "d157" angle of L112 L118
  measures "d158" radius of A78
  measures "d159" radius of A60
  measures "d160" radius of A79
  measures "d161" angle of L81 L108
  measures "d162" distance of P22 L92
  measures "d163" distance of P22 L96
  measures "d164" distance of P22 L110
  measures "d165" distance of L101 L118
  measures "d166" angle of L112 L113
  measures "d167" angle of L90 L109
  measures "d168" distance of A60.centre L92
  measures "d169" diameter of A74
  measures "d170" diameter of A77
  measures "d171" distance of L74.start P18
  measures "d172" distance of L74.start L75.end
  measures "d173" radius of A58
  measures "d174" radius of A52
  measures "d175" radius of A56
  measures "d176" angle of L78 L116
  measures "d177" radius of A57
  measures "d178" radius of A55
  measures "d179" radius of A75
  measures "d180" angle of L79 L107
  measures "d181" distance of P19 L117
  measures "d182" distance of P19 L85
  measures "d183" distance of P19 L80
  measures "d184" distance of L82 L116
  measures "d185" angle of L75 L78
  measures "d186" angle of L84 L86
  measures "d187" distance of A52.centre L117
  measures "d188" diameter of A62
  measures "d189" diameter of A76
  measures "d190" distance of P29 L65.start
  measures "d191" distance of L64.start L65.start
  measures "d192" radius of A45
  measures "d193" radius of A69
  measures "d194" radius of A50
  measures "d195" angle of L93 L94
  measures "d196" radius of A68
  measures "d197" radius of A44
  measures "d198" radius of A46
  measures "d199" angle of L62 L63
  measures "d200" distance of P31 L67
  measures "d201" distance of P31 L105
  measures "d202" distance of P31 L60
  measures "d203" distance of L77 L94
  measures "d204" angle of L93 L95
  measures "d205" angle of L73 L106
  measures "d206" distance of A44.centre L67
  measures "d207" diameter of A65
  measures "d208" diameter of A51
  measures "d211" diameter of A88
  measures "d212" diameter of A89
extrude "Extrude2" add sketch "Sketch2" along normal blind 20 contours A89 makes body 1
extrude "Extrude3" add sketch "Sketch2" along normal blind 20 separate body contours L120 L122 A88 A90 | L120 L122 A88 A90 | L120 L122 A88 A90 | L120 L122 A88 A90 makes body 2
extrude "Extrude6" add sketch "Sketch2" along normal blind 5 separate body contours L0 L1 A1 A3 L2 L4 A5 L5 A6 L6 A7 A8 L10 L11 L12 L14 L16 A13 A14 L18 L60 L61 A44 A45 L65 L72 A68 A69 | L1 A2 A3 L3 L62 A44 L63 L65 A46 L67 A49 L72 L73 A50 L74 A52 L76 A54 A55 L77 A57 A58 L80 L93 A69 L94 L103 L106 | L1 L5 L10 L11 L16 L20 L25 L26 L35 L40 L45 L47 L120 L122 A88 | L65 L67 L72 L77 L120 L121 L122 A88 | A5 L5 A8 L8 L9 A9 L11 A10 L15 L16 A12 A14 L17 L19 A16 L20 A17 L21 A18 A19 L25 L26 L27 L29 A38 L47 A39 L56 | L66 L71 L74 L82 L87 L92 L101 L102 L103 L115 L117 L119 L120 L121 L122 A88 | L74 A52 A53 A54 A55 A56 L77 L78 L79 L82 L84 A59 A60 L86 A63 L87 A75 L103 L105 A78 L107 L110 A82 A84 L114 L116 L117 L119 | L31 L32 L41 L55 L120 L122 A88 | L30 L31 L32 A22 L33 A24 L35 A25 L38 L39 L40 A28 A29 L41 A33 L43 A34 A40 A41 L51 L52 A42 L54 L55 L66 A47 A48 L68 | L31 A23 L34 A24 A42 A43 L55 L58 L66 A47 L69 L70 L71 L88 L89 A67 L91 A70 L96 L98 A71 L101 L102 A73 A83 L115 A85 A86 | A16 L20 A19 L23 L24 A20 L26 A21 L35 A26 A27 L40 A28 L41 L42 A30 A33 L44 L45 A37 A38 L46 L47 L48 A40 L49 L50 L57 | L81 L82 L85 A60 A61 A63 A64 L87 L90 L92 A72 L100 L101 L102 A73 A79 L108 A81 L109 L111 L112 A83 A84 L115 A86 L118 A87 L119 | A89 makes body 3
combine "Combine1" operation add target body 1 tool bodies 2 3
revolve "Revolve1" [rolled back] along angle 360
sketch "Sketch3" plane through (0, 0, 0) normal (0, 0, 1) x (1, 0, 0)
  line L0 (11.3, 66.9) -> (-11.34, 12.33)
  line L1 (11.32, 12.3313) -> (-11.3807, 66.9365)
  circle A0 centre (-0.02, 39.615) radius 25
  circle A1 centre (-0.02, 39.615) radius 50
  dimension "d209" = 50
  dimension "d210" = 100
  constraint midpoint L0 A0.centre
  constraint concentric A0 A1
  measures "d209" diameter of A0
  measures "d210" diameter of A1
